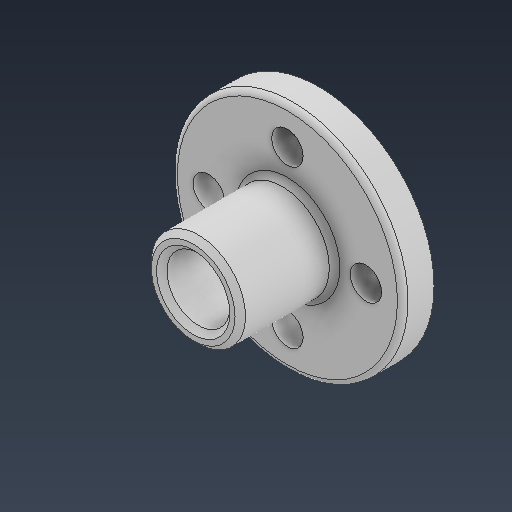
# Autodesk Inventor part: МУФТА НА ВАЛ
Saved by Autodesk Inventor 2026 (Build 300175000, 175)
## iProperties
Created: 2026-01-10
Part Number: МУФТА НА ВАЛ
Material: Типовые
Document SubType Name: Modeling
Designer: GameHD
Density: 1 g/cm^3
Appearance: По умолчанию
Author: GameHD
Autodesk Inventor part; units mm, degrees
ref_plane "YZ Plane" through (0, 0, 0) normal (1, 0, 0) x (0, 1, 0)
ref_plane "XZ Plane" through (0, 0, 0) normal (0, 1, 0) x (-1, 0, 0)
ref_plane "XY Plane" through (0, 0, 0) normal (0, 0, 1) x (1, 0, 0)
sketch "Эскиз1" plane through (0, 0, 0) normal (0, 0, 1) x (1, 0, 0)
  circle A0 centre (0, 0) radius 11
  circle A1 centre (0, 0) radius 7.5
  circle A2 centre (-7.5, 0) radius 1.5
  circle A3 centre (0, -7.5) radius 1.5
  circle A4 centre (7.5, 0) radius 1.5
  circle A5 centre (0, 7.5) radius 1.5
  circle A6 centre (0, 0) radius 3
  dimension "d1" = 15
  dimension "d0" = 22
  dimension "d2" = 3
  dimension "d5" = 360
  dimension "d7" = 6
  constraints: 6 centre point, 5 coincident, 1 horizontal alignment, 11 other
  measures "d0" diameter of A0
  measures "d2" diameter of A2
  measures "d7" diameter of A6
extrude "Выдавливание1" add sketch "Эскиз1" along normal blind 3 contours A0 | A4 A1 A3 A2 A5
sketch "Эскиз2" plane through (0, 0, 3) normal (0, 0, 1) x (1, 0, 0)
  circle A0 centre (0, 0) radius 4.5
  circle A1 centre (0, 0) radius 11 projected
  circle A2 centre (0, 7.5) radius 1.5 projected
  circle A3 centre (-7.5, 0) radius 1.5 projected
  circle A4 centre (0, -7.5) radius 1.5 projected
  circle A5 centre (0, 0) radius 3 projected
  circle A6 centre (7.5, 0) radius 1.5 projected
  dimension "d10" = 9
  constraints: 1 centre point, 1 coincident
  measures "d10" diameter of A0
extrude "Выдавливание2" add sketch "Эскиз2" along normal blind 9 contours A0
fillet "Сопряжение1" radius 0.5 2 edges at (-11, 0, 3) (-4.5, 0, 3)
chamfer "Фаска1" distance 0.5 angle 45 2 edges at (-4.5, 0, 12) (-3, 0, 12)
